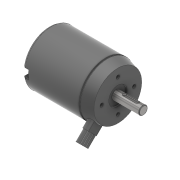
# Autodesk Inventor part: Flipsky_5065-270KV
Saved by Autodesk Inventor 2020.3 (Build 243373000, 373)
## iProperties
Created: 2022-08-06
Part Number: Flipsky_5065-270KV
Material: Steel, Mild
Document SubType Name: Modeling
Designer: User
Density: 7.85 g/cm^3
Appearance: Smooth - Black
Mass: 934.871 g
Surface Area: 150.846 cm^2
Volume: 119.092 cm^3
Author: User
Autodesk Inventor part; units mm, degrees
ref_plane "YZ Plane" through (0, 0, 0) normal (1, 0, 0) x (0, 1, 0)
sketch "Sketch1" plane through (0, 0, 0) normal (0, 0, 1) x (1, 0, 0)
  line L0 (0, 0) -> (0, 24.75)
  line L1 (0, 24.75) -> (53.3, 24.75)
  line L2 (53.3, 24.75) -> (63, 22.11)
  line L3 (63, 22.11) -> (63, 0)
  line L4 (63, 0) -> (0, 0)
  line L5 (52.8, 24.75) -> (51.8, 24.75)
  line L6 (51.8, 24.75) -> (51.8, 21.75)
  line L7 (51.8, 21.75) -> (52.8, 21.75)
  line L8 (52.8, 21.75) -> (52.8, 24.75)
  dimension "d0" = 49.5
  dimension "d1" = 63
  dimension "d2" = 9.7
  dimension "d3" = 44.22
  dimension "d40" = 0.5
  dimension "d41" = 1
  dimension "d42" = 3
  constraints: 18 end point, 3 parallel, 3 perpendicular, 1 horizontal, 1 point on line, 1 vertical
  measures "d0" diameter of L1 L4
  measures "d1" distance between parallel lines of L0 L3
  measures "d2" distance from line of L3 L1.end
  measures "d3" diameter of L2.end L4
  measures "d40" distance from line of L8 L1.end
  measures "d41" distance of L6.end L7.end
  measures "d42" distance of L5.end L6.end
revolve "Revolution1" add sketch "Sketch1" angle 360 about axis through (63, 0, 0) along (-1, 0, 0) contours L0 L1 L6 L7 L8 L2 L3 L4
sketch "Sketch2" plane through (0, 0, 0) normal (-1, 0, 0) x (0, 0, 1)
  circle A0 centre (0, 0) radius 7
  circle A1 centre (0, 0) radius 4.025
  point P0 (0, 0)
  dimension "d5" = 14
  dimension "d31" = 8.05
  constraints: 2 centre point, 2 coincident
  measures "d5" diameter of A0
  measures "d31" diameter of A1
extrude "Extrusion1" add sketch "Sketch2" along normal blind 4 separate body
sketch "Sketch3" plane through (63, 0, 0) normal (1, 0, 0) x (0, 0, -1)
  circle A0 centre (0, 0) radius 4
  dimension "d8" = 8
  constraints: 1 centre point, 1 coincident
  measures "d8" diameter of A0
extrude "Extrusion2" add sketch "Sketch3" along normal blind 23.7 separate body
sketch "Sketch5" plane through (63, 0, 0) normal (1, 0, 0) x (0, 0, -1)
  circle A0 centre (0, 0) radius 4 construction
  circle A1 centre (0, 0) radius 15 construction
  point P0 (15, 0)
  point P1 (0, 15)
  point P2 (-15, 0)
  point P3 (0, -15)
  dimension "d19" = 30
  dimension "d22" = 360
  constraints: 2 horizontal alignment, 1 coincident, 7 other
hole "Hole1" at (63, 0, -15) at (63, 15, 0) at (63, 0, 15) at (63, -15, 0) direction (-1, 0, 0) diameter 3.242 depth 6 tip angle 118 bodies 1 thread size "M4x0.7" class "6H" standard "ISO Metric profile"
sketch "Sketch6" plane through (0, 0, 0) normal (-1, 0, 0) x (0, 0, 1)
  circle A0 centre (0, 0) radius 4
  point P0 (0, 0)
  dimension "d32" = 8
  constraints: 1 centre point, 1 coincident
  measures "d32" diameter of A0
extrude "Extrusion4" add sketch "Sketch6" along normal blind 4 bodies 3
sketch "Sketch7" plane through (0, 0, 0) normal (-1, 0, 0) x (0, 0, 1)
  line L0 (27.4626, 4) -> (12.15, 4)
  arc A0 (12.15, 4) -> (12.15, -4) centre (12.15, 0) ccw
  line L1 (12.15, -4) -> (27.4626, -4)
  line L2 (27.4626, -4) -> (27.4626, 4)
  circle A1 centre (0, 0) radius 4.025 construction
  line L3 (-28.0701, 4) -> (-12.15, 4)
  arc A2 (-12.15, -4) -> (-12.15, 4) centre (-12.15, 0) ccw
  line L4 (-12.15, -4) -> (-28.0701, -4)
  line L5 (-28.0701, 4) -> (-28.0701, -4)
  point P0 (0, 0)
  dimension "d35" = 8
  dimension "d36" = 16.3
  dimension "d37" = 12.15
  constraints: 12 end point, 4 point on circle, 4 tangent, 3 horizontal, 2 centre point, 2 collinear, 1 horizontal alignment, 1 parallel, 1 perpendicular, 1 vertical
  measures "d35" distance between parallel lines of L1 L0
  measures "d37" distance of A0.centre point (0, 0)
extrude "Extrusion5" cut sketch "Sketch7" against normal blind 5 bodies 1
sketch "Sketch8" plane through (63, 0, 0) normal (1, 0, 0) x (0, 0, -1)
  circle A0 centre (0, 0) radius 4 projected
  circle A1 centre (0, 0) radius 8.5
  dimension "d43" = 17
  constraints: 1 centre point
  measures "d43" diameter of A1
extrude "Extrusion6" cut sketch "Sketch8" against normal blind 1.5 bodies 1
fillet "Fillet2" radius 0.2 2 edges at (-4, 0, -4.025) (-4, 0, -4)
fillet "Fillet3" radius 0.5 1 edges at (-4, 0, -7)
chamfer "Chamfer1" distance 1.5 distance2 1 1 edges at (0, -24.75, 0) measured on face at (0.5, -24.75, 0)
chamfer "Chamfer2" distance 1.5 distance2 1 2 edges at (0, 18.8622, 16.0244) (0, 18.8622, -16.0244) measured on face at (0.5, 18.8622, 16.0244) measured on face at (0.5, 18.8622, -16.0244)
ref_plane "Work Plane2" through (63, 4, 0) normal (0, 1, 0) x (-1, 0, 0)
sketch "Sketch9" plane through (63, 4, 0) normal (0, 1, 0) x (-1, 0, 0)
  line L0 (-6.2, 0) -> (-18.2, 0) construction
  line L1 (-6.2, 1.5) -> (-18.2, 1.5)
  line L2 (-18.2, -1.5) -> (-6.2, -1.5)
  arc A0 (-6.2, -1.5) -> (-6.2, 1.5) centre (-6.2, 0) ccw
  arc A1 (-18.2, 1.5) -> (-18.2, -1.5) centre (-18.2, 0) ccw
  line L3 (-23.7, 4) -> (-23.7, -4) construction
  line L4 (0, 4) -> (0, -4) construction
  point P0 (63, 0)
  point P1 (-12.2, 0)
  point P2 (-19.7, 0)
  point P3 (0, 0)
  dimension "d54" = 4
  dimension "d55" = 12
  dimension "d56" = 3
  constraints: 8 end point, 5 point on circle, 4 tangent, 2 centre point, 2 midpoint, 1 horizontal, 1 horizontal alignment, 1 parallel
  measures "d54" distance from line of L3 point (-19.7, 0)
  measures "d55" distance of L0.start L0.end
  measures "d56" distance between parallel lines of L2 L1
extrude "Extrusion7" cut sketch "Sketch9" along normal mid plane 3 bodies 3
combine bodies "Combine1" operation type add bodies to combine 1 2
combine bodies "Combine2" operation type add bodies to combine 1 3
chamfer "Chamfer3" distance 0.5 angle 45 1 edges at (86.7, 0, 4)
ref_plane "Work Plane4" through (53.05, -17.5009, 17.5009) normal (0, 0.7071068, -0.7071068) x (-1, 0, 0)
ref_plane "Work Plane3" through (0, 0, 0) normal (0, 0.7071068, -0.7071068) x (-1, 0, 0)
sketch "Sketch10" plane through (53.05, -17.5009, 17.5009) normal (0, 0.7071068, -0.7071068) x (-1, 0, 0)
  line L0 (-4.85, 4.9) -> (-4.85, -4.9) construction
  line L1 (-7.45, 4.9) -> (-7.45, -4.9)
  line L2 (-2.25, -4.9) -> (-2.25, 4.9)
  arc A0 (-2.25, 4.9) -> (-7.45, 4.9) centre (-4.85, 4.9) ccw
  arc A1 (-7.45, -4.9) -> (-2.25, -4.9) centre (-4.85, -4.9) ccw
  line L3 (-9.95, 22.11) -> (-9.95, -22.11) construction
  line L4 (0.25, 24.75) -> (0.25, -24.75) construction
  point P0 (53.05, 0)
  point P1 (-4.85, 0)
  point P2 (0.25, 0)
  dimension "d62" = 2.5
  dimension "d63" = 2.5
  dimension "d64" = 15
  constraints: 8 end point, 4 point on circle, 4 tangent, 2 centre point, 2 midpoint, 1 horizontal alignment, 1 parallel, 1 vertical
  measures "d62" distance between parallel lines of L3 L1
  measures "d63" distance between parallel lines of L4 L2
extrude "Extrusion8" add sketch "Sketch10" along normal mid plane 10 bodies 1
sketch "Sketch11" plane through (53.05, -21.0364, 21.0364) normal (0, -0.7071068, 0.7071068) x (1, 0, 0)
  arc A0 (2.25, -4.9) -> (7.45, -4.9) centre (4.85, -4.9) ccw construction
  arc A1 (7.45, 4.9) -> (2.25, 4.9) centre (4.85, 4.9) ccw construction
  circle A2 centre (4.85, 5.1663) radius 1.75
  circle A3 centre (4.85, 1.6663) radius 1.75
  circle A4 centre (4.85, -1.8337) radius 1.75
  circle A5 centre (4.85, -5.3337) radius 1.75
  point P0 (-53.05, 0)
  point P1 (4.85, -3.5837)
  point P2 (4.85, -0.0837)
  point P3 (4.85, 3.4163)
  dimension "d67" = 3.5
  dimension "d68" = 3.5
  constraints: 5 equal radius, 4 centre point, 4 vertical alignment
  measures "d67" diameter of A2
  measures "d68" distance of A4.centre A3.centre
extrude "Extrusion9" add sketch "Sketch11" along normal blind 10 bodies 1
equation "\"d63\" = d62"
body "Solid1"
